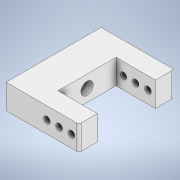
# Autodesk Inventor part: LowerJawLoadCell
Saved by Autodesk Inventor 2022 (Build 260153000, 153)
## iProperties
Created: 2021-11-03
Part Number: LowerJawLoadCell
Material: Plástico ABS
Document SubType Name: Modeling
Designer: JK
Density: 1.06 g/cm^3
Appearance: Suave - Blanco
Author: JK
Autodesk Inventor part; units mm, degrees
ref_plane "YZ Plane" through (0, 0, 0) normal (1, 0, 0) x (0, 1, 0)
ref_plane "XZ Plane" through (0, 0, 0) normal (0, 1, 0) x (-1, 0, 0)
ref_plane "XY Plane" through (0, 0, 0) normal (0, 0, 1) x (1, 0, 0)
sketch "Boceto1" plane through (0, 0, 0) normal (0, 1, 0) x (-1, 0, 0)
  line L0 (-38.575, 38.575) -> (38.575, 38.575)
  line L1 (38.575, 38.575) -> (38.575, -38.575)
  line L2 (38.575, -38.575) -> (-38.575, -38.575)
  line L3 (-38.575, -38.575) -> (-38.575, 38.575)
  line L4 (-38.575, 38.575) -> (38.575, -38.575) construction
  line L5 (38.575, 38.575) -> (-38.575, -38.575) construction
  circle A0 centre (17, 10) radius 2.7
  circle A1 centre (17, -10) radius 2.7
  circle A2 centre (-17, -10) radius 2.7
  circle A3 centre (-17, 10) radius 2.7
  point P0 (0, 0)
  dimension "d0" = 77.15
  dimension "d1" = 77.15
  dimension "d2" = 5.4
  dimension "d3" = 10
  dimension "d4" = 10
  dimension "d5" = 17
  dimension "d6" = 17
  constraints: 12 end point, 4 centre point, 3 equal radius, 2 horizontal alignment, 2 midpoint, 2 parallel, 2 vertical alignment, 1 horizontal, 1 perpendicular
  measures "d0" distance of L1.end L2.end
  measures "d1" distance of L0.end L1.end
  measures "d2" diameter of A0
  measures "d3" vertical distance of point (0, 0) A0.centre
  measures "d4" vertical distance of point (0, 0) A1.centre
  measures "d5" horizontal distance of point (0, 0) A0.centre
  measures "d6" horizontal distance of point (0, 0) A3.centre
extrude "Extrusión1" add sketch "Boceto1" along normal blind 20
sketch "Boceto2" plane through (0, 20, 0) normal (0, 1, 0) x (1, 0, 0)
  line L0 (-38.575, -38.575) -> (38.575, -38.575) projected
  line L1 (38.575, -38.575) -> (70.575, -38.575)
  line L2 (70.575, -38.575) -> (70.575, -23.575)
  line L3 (70.575, -23.575) -> (38.575, -23.575)
  line L4 (38.575, -23.575) -> (38.575, -38.575)
  line L5 (38.575, 38.575) -> (-38.575, 38.575) projected
  line L6 (38.575, 38.575) -> (70.575, 38.575)
  line L7 (70.575, 38.575) -> (70.575, 23.575)
  line L8 (70.575, 23.575) -> (38.575, 23.575)
  line L9 (38.575, 23.575) -> (38.575, 38.575)
  point P0 (0, 0)
  dimension "d9" = 32
  dimension "d10" = 15
  constraints: 16 end point, 4 parallel, 2 horizontal, 2 perpendicular, 1 collinear, 1 point on line
  measures "d9" distance between parallel lines of L4 L2
  measures "d10" distance between parallel lines of L3 L1
extrude "Extrusión2" add sketch "Boceto2" against normal up to surface (20 mm away)
sketch "Boceto3" plane through (-38.575, 0, 38.575) normal (0, 0, 1) x (1, 0, 0)
  circle A0 centre (103.15, 10) radius 2.7
  circle A1 centre (93.15, 10) radius 2.7
  line L0 (109.15, 20) -> (109.15, 0) projected
  circle A2 centre (83.15, 10) radius 2.7
  point P0 (38.575, 0)
  dimension "d13" = 5.4
  dimension "d14" = 6
  dimension "d15" = 10
  dimension "d34" = 10
  constraints: 3 centre point, 2 equal radius
  measures "d13" diameter of A1
  measures "d14" distance from line of L0 A0.centre
  measures "d15" distance of A0.centre A1.centre
  measures "d34" distance of A2.centre A1.centre
extrude "Extrusión3" cut sketch "Boceto3" against normal through all
fillet "Empalme2" radius 4.635 2 edges at (-38.575, 10, 38.575) (-38.575, 10, -38.575)
fillet "Empalme3" radius 2 2 edges at (70.575, 10, -38.575) (70.575, 10, 38.575)
sketch "Boceto5" plane through (0, 20, 0) normal (0, 1, 0) x (1, 0, 0)
  line L0 (-29.2306, -22.0337) -> (29.2306, -22.0337)
  line L1 (29.2306, -22.0337) -> (29.2306, 22.0337)
  line L2 (29.2306, 22.0337) -> (-29.2306, 22.0337)
  line L3 (-29.2306, 22.0337) -> (-29.2306, -22.0337)
  line L4 (-29.2306, -22.0337) -> (29.2306, 22.0337) construction
  line L5 (29.2306, -22.0337) -> (-29.2306, 22.0337) construction
  point P0 (0, 0)
  constraints: 12 end point, 2 midpoint, 2 parallel, 1 horizontal, 1 perpendicular
extrude "Extrusión5" add sketch "Boceto5" against normal up to surface (20 mm away)
sketch "Boceto6" plane through (-38.575, 0, -33.94) normal (-1, 0, 0) x (0, 0, 1)
  line L0 (-23.6354, 28.4555) -> (91.5154, 28.4555)
  line L1 (91.5154, 28.4555) -> (91.5154, -11.4044)
  line L2 (91.5154, -11.4044) -> (-23.6354, -11.4044)
  line L3 (-23.6354, -11.4044) -> (-23.6354, 28.4555)
  line L4 (-23.6354, 28.4555) -> (91.5154, -11.4044) construction
  line L5 (91.5154, 28.4555) -> (-23.6354, -11.4044) construction
  point P0 (33.94, 0)
  point P1 (33.94, 8.5256)
  constraints: 12 end point, 2 midpoint, 2 parallel, 1 horizontal, 1 perpendicular
extrude "Extrusión6" cut sketch "Boceto6" against normal blind 50
sketch "Boceto7" plane through (11.425, 0, -33.94) normal (-1, 0, 0) x (0, 0, 1)
  line L0 (59.44, 3.5) -> (8.44, 3.5)
  line L1 (8.44, 3.5) -> (8.44, 16.5)
  line L2 (8.44, 16.5) -> (59.44, 16.5)
  line L3 (59.44, 16.5) -> (59.44, 3.5)
  line L4 (59.44, 3.5) -> (8.44, 16.5) construction
  line L5 (8.44, 3.5) -> (59.44, 16.5) construction
  line L6 (72.515, 0) -> (-4.635, 0) projected
  point P0 (33.94, 0)
  point P1 (33.94, 10)
  point P2 (33.94, 10)
  point P3 (33.94, 0)
  dimension "d39" = 13
  dimension "d40" = 51
  dimension "d41" = 3.5
  constraints: 12 end point, 4 midpoint, 2 parallel, 1 horizontal, 1 perpendicular, 1 vertical alignment
  measures "d39" distance of L0.end L1.end
  measures "d40" distance of L0.start L0.end
  measures "d41" distance between parallel lines of L6 L0
extrude "Extrusión7" cut sketch "Boceto7" against normal blind 4
sketch "Boceto8" plane through (15.425, 0, -33.94) normal (-1, 0, 0) x (0, 0, 1)
  circle A0 centre (33.94, 10) radius 3.5
  point P0 (33.94, 0)
  dimension "d44" = 7
  constraints: 1 centre point
  measures "d44" diameter of A0
extrude "Extrusión8" cut sketch "Boceto8" against normal through all
sketch "Boceto9" plane through (38.575, 0, 23.575) normal (1, 0, 0) x (0, 0, -1)
  circle A0 centre (23.575, 10) radius 3.5 projected
  circle A1 centre (23.575, 10) radius 5
  point P0 (23.575, 0)
  dimension "d47" = 10
  constraints: 1 centre point, 1 coincident
  measures "d47" diameter of A1
extrude "Extrusión9" cut sketch "Boceto9" against normal blind 5 contours A0 | A1
sketch "Boceto4" plane through (0, 20, 0) normal (0, 1, 0) x (1, 0, 0)
  line L0 (53.225, -32.695) -> (61.325, -32.695)
  line L1 (61.325, -32.695) -> (61.325, -28.455)
  line L2 (61.325, -28.455) -> (53.225, -28.455)
  line L3 (53.225, -28.455) -> (53.225, -32.695)
  line L4 (53.225, -32.695) -> (61.325, -28.455) construction
  line L5 (61.325, -32.695) -> (53.225, -28.455) construction
  line L6 (57.275, -38.575) -> (51.875, -38.575) projected
  point P0 (0, 0)
  point P1 (57.275, -30.575)
  dimension "d21" = 8.1
  dimension "d23" = 1.35
  dimension "d24" = 8
  dimension "d25" = 4.24
  constraints: 12 end point, 2 midpoint, 2 parallel, 1 horizontal, 1 perpendicular
  measures "d21" distance between parallel lines of L3 L1
  measures "d23" distance from line of L6.end L3
  measures "d24" distance from line of L6 point (57.275, -30.575)
  measures "d25" distance of L2.end L0.start
